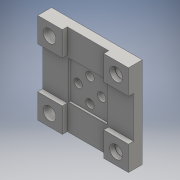
# Autodesk Inventor part: RotatorBottom
Saved by Autodesk Inventor 2016 (Build 200138000, 138)
## iProperties
Created: 2016-03-27
Part Number: RotatorBottom
Material: Generic
Document SubType Name: Modeling
Designer: mkepler
Density: 1 g/cm^3
Appearance: Default
Author: mkepler
Autodesk Inventor part; units mm, degrees
ref_plane "YZ Plane" through (0, 0, 0) normal (1, 0, 0) x (0, 1, 0)
ref_plane "XZ Plane" through (0, 0, 0) normal (0, 1, 0) x (-1, 0, 0)
ref_plane "XY Plane" through (0, 0, 0) normal (0, 0, 1) x (1, 0, 0)
sketch "Sketch2" plane through (0, 0, 0) normal (0, 1, 0) x (-1, 0, 0)
  line L0 (0, 0) -> (46, 0)
  line L1 (46, 0) -> (46, -46)
  line L2 (46, -46) -> (0, -46)
  line L3 (0, -46) -> (0, 0)
  dimension "d0" = 46
  dimension "d1" = 46
  constraints: 8 end point, 2 parallel, 1 horizontal, 1 perpendicular
  measures "d0" distance of L1.end L2.end
  measures "d1" distance of L0.end L1.end
extrude "Extrusion1" add sketch "Sketch2" along normal blind 3.5
sketch "Sketch6" plane through (0, 0, 0) normal (0, -1, 0) x (1, 0, 0)
  line L0 (-13.25, -13.25) -> (-32.75, -13.25)
  line L1 (-32.75, -13.25) -> (-32.75, -32.75)
  line L2 (-32.75, -32.75) -> (-13.25, -32.75)
  line L3 (-13.25, -32.75) -> (-13.25, -13.25)
  line L4 (-46, -46) -> (0, -46) projected
  line L5 (0, 0) -> (0, -46) projected
  line L6 (-46, -46) -> (-46, 0) projected
  line L7 (0, 0) -> (-46, 0)
  line L8 (-46, 0) -> (-46, -46)
  line L9 (-46, -46) -> (0, -46)
  line L10 (0, -46) -> (0, 0)
  dimension "d41" = 13.25
  dimension "d42" = 13.25
  dimension "d43" = 13.25
  dimension "d44" = 13.25
  constraints: 16 end point, 4 parallel, 2 horizontal, 2 perpendicular
  measures "d41" distance between parallel lines of L7 L0
  measures "d42" distance between parallel lines of L3 L5
  measures "d43" distance between parallel lines of L4 L2
  measures "d44" distance between parallel lines of L6 L1
extrude "Extrusion3" add sketch "Sketch6" along normal blind 1
sketch "Sketch7" plane through (0, -1, 0) normal (0, -1, 0) x (1, 0, 0)
  circle A0 centre (-6, -40) radius 3.25
  line L0 (-46, -46) -> (0, -46) projected
  line L1 (0, -46) -> (0, 0) projected
  circle A1 centre (-40, -40) radius 3.25
  line L2 (-46, 0) -> (-46, -46) projected
  circle A2 centre (-40, -6) radius 3.25
  line L3 (0, 0) -> (-46, 0) projected
  circle A3 centre (-6, -6) radius 3.25
  dimension "d26" = 6.5
  dimension "d27" = 6
  dimension "d28" = 6
  dimension "d29" = 6.5
  dimension "d30" = 6
  dimension "d31" = 6.5
  dimension "d32" = 6
  dimension "d33" = 6.5
  dimension "d45" = 6
  dimension "d46" = 6
  dimension "d47" = 6
  dimension "d48" = 6
  constraints: 4 centre point
  measures "d26" diameter of A0
  measures "d27" distance from line of L0 A0.centre
  measures "d28" distance from line of L1 A0.centre
  measures "d29" diameter of A1
  measures "d30" distance from line of L2 A1.centre
  measures "d31" diameter of A2
  measures "d32" distance from line of L3 A2.centre
  measures "d33" diameter of A3
  measures "d45" distance from line of L0 A1.centre
  measures "d46" distance from line of L2 A2.centre
  measures "d47" distance from line of L1 A3.centre
  measures "d48" distance from line of L3 A3.centre
hole "Hole2" at (-6, -1, -6) at (-6, -1, -40) at (-40, -1, -40) at (-40, -1, -6) direction (0, 1, 0) diameter 6.5 depth 9
sketch "Sketch8" plane through (0, 0, 0) normal (0, -1, 0) x (1, 0, 0)
  line L0 (-32.75, -13.25) -> (-13.25, -13.25) projected
  line L1 (-23, -13.25) -> (-23, -32.75)
  line L2 (-32.75, -32.75) -> (-13.25, -32.75) projected
  line L3 (-23, -23) -> (-11, -23)
  circle A0 centre (-17, -23) radius 2.125
  circle A1 centre (-23, -17) radius 2.125
  circle A2 centre (-23, -29) radius 2.125
  circle A3 centre (-29, -23) radius 2.125
  point P0 (0, 0)
  dimension "d49" = 4.25
  dimension "d50" = 6
  dimension "d51" = 4.25
  dimension "d52" = 6
  dimension "d53" = 4.25
  dimension "d54" = 6
  dimension "d55" = 4.25
  dimension "d56" = 6
  constraints: 4 centre point, 4 end point, 4 midpoint, 2 point on line, 1 horizontal
  measures "d49" diameter of A0
  measures "d50" distance of L3.start A0.centre
  measures "d51" diameter of A1
  measures "d52" distance of L3.start A1.centre
  measures "d53" diameter of A2
  measures "d54" distance of L3.start A2.centre
  measures "d55" diameter of A3
  measures "d56" distance of A3.centre L3.start
hole "Hole3" at (-29, 0, -23) at (-23, 0, -17) at (-23, 0, -29) at (-17, 0, -23) direction (0, 1, 0) diameter 4.25 end through all
sketch "Sketch9" plane through (0, -1, 0) normal (0, -1, 0) x (1, 0, 0)
  line L0 (0, 0) -> (-46, 0) projected
  line L1 (0, 0) -> (-12.5, 0)
  line L2 (-12.5, 0) -> (-12.5, -12.5)
  line L3 (-12.5, -12.5) -> (0, -12.5)
  line L4 (0, -12.5) -> (0, 0)
  line L5 (-46, -46) -> (0, -46) projected
  line L6 (0, -46) -> (-12.5, -46)
  line L7 (-12.5, -46) -> (-12.5, -33.5)
  line L8 (-12.5, -33.5) -> (0, -33.5)
  line L9 (0, -33.5) -> (0, -46)
  line L10 (-46, -46) -> (-33.5, -46)
  line L11 (-33.5, -46) -> (-33.5, -33.5)
  line L12 (-33.5, -33.5) -> (-46, -33.5)
  line L13 (-46, -33.5) -> (-46, -46)
  circle A0 centre (-40, -40) radius 3.25 projected
  circle A1 centre (-40, -40) radius 3.25
  circle A2 centre (-40, -6) radius 3.25 projected
  circle A3 centre (-40, -6) radius 3.25
  circle A4 centre (-6.25, -40) radius 3.25
  circle A5 centre (-6.25, -6) radius 3.25
  line L14 (-46, 0) -> (-33.5, 0)
  line L15 (-33.5, 0) -> (-33.5, -12.5)
  line L16 (-33.5, -12.5) -> (-46, -12.5)
  line L17 (-46, -12.5) -> (-46, 0)
  dimension "d66" = 12.5
  dimension "d67" = 12.5
  dimension "d68" = 12.5
  dimension "d69" = 12.5
  dimension "d70" = 12.5
  dimension "d71" = 12.5
  dimension "d72" = 6.5
  dimension "d73" = 6.5
  dimension "d74" = 6.5
  dimension "d77" = 12.5
  dimension "d78" = 12.5
  constraints: 32 end point, 8 parallel, 4 centre point, 4 horizontal, 4 perpendicular, 2 coincident
  measures "d66" distance of L3.end L2.end
  measures "d67" distance of L2.end L1.end
  measures "d68" distance of L7.end L8.end
  measures "d69" distance of L6.end L7.end
  measures "d70" distance of L12.end L11.end
  measures "d71" distance of L11.end L10.end
  measures "d72" diameter of A3
  measures "d73" diameter of A4
  measures "d74" diameter of A5
  measures "d77" distance of L15.end L16.end
  measures "d78" distance of L14.end L15.end
extrude "Extrusion4" add sketch "Sketch9" along normal blind 2.5
body "Solid1"
